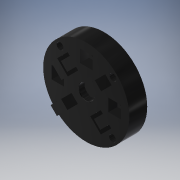
# Autodesk Inventor part: amt_socket
Saved by Autodesk Inventor 2019 (Build 230136000, 136)
## iProperties
Created: 2024-04-30
Part Number: amt_socket
Material: Acetalharz, Schwarz
Document SubType Name: Modeling
Designer: nic
Density: 1.425 g/cm^3
Appearance: Glatt - Schwarz
Author: nic
Autodesk Inventor part; units mm, degrees
ref_plane "YZ Plane" through (0, 0, 0) normal (1, 0, 0) x (0, 1, 0)
ref_plane "XZ Plane" through (0, 0, 0) normal (0, 1, 0) x (-1, 0, 0)
ref_plane "XY Plane" through (0, 0, 0) normal (0, 0, 1) x (1, 0, 0)
sketch "Skizze1" plane through (0, 0, 0) normal (0, 0, 1) x (1, 0, 0)
  circle A0 centre (0, 0) radius 14.5
  circle A1 centre (0, 0) radius 9.55 construction
  circle A2 centre (9.55, 0) radius 1.5
  circle A3 centre (-9.55, 0) radius 1.5
  circle A4 centre (0, 9.55) radius 1.5
  dimension "d0" = 29
  dimension "d1" = 19.1
  dimension "d2" = 3
  dimension "d3" = 3
  dimension "d4" = 3
  constraints: 5 centre point, 3 point on circle, 2 coincident
  measures "d0" diameter of A0
  measures "d1" diameter of A1
  measures "d2" diameter of A2
  measures "d3" diameter of A3
  measures "d4" diameter of A4
extrude "Extrusion1" add sketch "Skizze1" along normal blind 6
sketch "Skizze2" plane through (0, 0, 6) normal (0, 0, 1) x (1, 0, 0)
  circle A0 centre (0, 0) radius 5.6
  dimension "d7" = 11.2
  constraints: 1 centre point, 1 coincident
  measures "d7" diameter of A0
extrude "Extrusion2" cut sketch "Skizze2" against normal blind 5
sketch "Skizze3" plane through (0, 0, 1) normal (0, 0, 1) x (1, 0, 0)
  circle A0 centre (0, 0) radius 5.6 projected
  circle A1 centre (0, 0) radius 1.5
  dimension "d10" = 3
  constraints: 1 centre point, 1 coincident
  measures "d10" diameter of A1
extrude "Extrusion3" cut sketch "Skizze3" against normal through all contours A1
sketch "Skizze4" plane through (0, 0, 6) normal (0, 0, 1) x (1, 0, 0)
  circle A0 centre (0, 9.55) radius 1.5 construction
  circle A1 centre (9.55, 0) radius 1.5 construction
  circle A2 centre (-9.55, 0) radius 1.5 construction
  line L0 (-2.85, 12.4) -> (2.85, 12.4)
  line L1 (2.85, 12.4) -> (2.85, 6.7)
  line L2 (2.85, 6.7) -> (-2.85, 6.7)
  line L3 (-2.85, 6.7) -> (-2.85, 12.4)
  line L4 (-2.85, 12.4) -> (2.85, 6.7) construction
  line L5 (2.85, 12.4) -> (-2.85, 6.7) construction
  line L6 (-12.4, 2.85) -> (-6.7, 2.85)
  line L7 (-6.7, 2.85) -> (-6.7, -2.85)
  line L8 (-6.7, -2.85) -> (-12.4, -2.85)
  line L9 (-12.4, -2.85) -> (-12.4, 2.85)
  line L10 (-12.4, 2.85) -> (-6.7, -2.85) construction
  line L11 (-6.7, 2.85) -> (-12.4, -2.85) construction
  line L12 (6.7, 2.85) -> (12.4, 2.85)
  line L13 (12.4, 2.85) -> (12.4, -2.85)
  line L14 (12.4, -2.85) -> (6.7, -2.85)
  line L15 (6.7, -2.85) -> (6.7, 2.85)
  line L16 (6.7, 2.85) -> (12.4, -2.85) construction
  line L17 (12.4, 2.85) -> (6.7, -2.85) construction
  point P0 (0, 0)
  point P1 (9.55, 0)
  dimension "d13" = 5.7
  dimension "d14" = 5.7
  dimension "d15" = 5.7
  dimension "d16" = 5.7
  dimension "d17" = 5.7
  dimension "d18" = 5.7
  constraints: 36 end point, 6 midpoint, 6 parallel, 3 horizontal, 3 perpendicular
  measures "d13" distance of L1.end L2.end
  measures "d14" distance of L0.end L1.end
  measures "d15" distance of L7.end L8.end
  measures "d16" distance of L6.end L7.end
  measures "d17" distance of L13.end L14.end
  measures "d18" distance of L12.end L13.end
extrude "Extrusion4" cut sketch "Skizze4" against normal blind 3
sketch "Skizze5" plane through (0, 0, 6) normal (0, 0, 1) x (1, 0, 0)
  circle A0 centre (0, 0) radius 5.6 projected
  line L0 (0, -5.6) -> (0, -8.2) construction
  circle A1 centre (0, -8.2) radius 1.45
  dimension "d21" = 2.6
  dimension "d22" = 2.9
  constraints: 2 end point, 1 centre point, 1 coincident, 1 vertical, 1 vertical alignment, 1 other
  measures "d21" distance of L0.start L0.end
  measures "d22" diameter of A1
hole "Bohrung1" at (0, -8.2, 6) direction (0, 0, -1) diameter 2.9 end through all countersink diameter 6 countersink angle 90
sketch "Skizze6" plane through (0, 0, 6) normal (0, 0, 1) x (1, 0, 0)
  circle A0 centre (-8.8221, 9.0078) radius 2.6 construction
  circle A1 centre (-8.8221, 9.0078) radius 1.15
  circle A2 centre (-9.0078, -8.8221) radius 1.15
  circle A3 centre (8.8221, -9.0078) radius 1.15
  circle A4 centre (9.0078, 8.8221) radius 1.15
  point P0 (0, 0)
  dimension "d30" = 2.3
  dimension "d33" = 360
  constraints: 4 centre point, 1 coincident, 9 other
  measures "d30" diameter of A1
extrude "Extrusion5" cut sketch "Skizze6" against normal through all
sketch "Skizze7" plane through (0, 0, 6) normal (0, 0, 1) x (1, 0, 0)
  line L0 (-6.3847, -8.3956) -> (-2.8458, -4.8634)
  line L1 (-2.8458, -4.8634) -> (-4.9651, -2.7401)
  line L2 (-4.9651, -2.7401) -> (-8.504, -6.2723)
  line L3 (-8.504, -6.2723) -> (-6.3847, -8.3956)
  line L4 (-6.3847, -8.3956) -> (-4.9651, -2.7401) construction
  line L5 (-2.8458, -4.8634) -> (-8.504, -6.2723) construction
  line L6 (2.7401, -4.9651) -> (6.2723, -8.504)
  line L7 (6.2723, -8.504) -> (8.3956, -6.3847)
  line L8 (8.3956, -6.3847) -> (4.8634, -2.8458)
  line L9 (4.8634, -2.8458) -> (2.7401, -4.9651)
  line L10 (4.9651, 2.7401) -> (8.504, 6.2723)
  line L11 (8.504, 6.2723) -> (6.3847, 8.3956)
  line L12 (6.3847, 8.3956) -> (2.8458, 4.8634)
  line L13 (2.8458, 4.8634) -> (4.9651, 2.7401)
  line L14 (-2.7401, 4.9651) -> (-6.2723, 8.504)
  line L15 (-6.2723, 8.504) -> (-8.3956, 6.3847)
  line L16 (-8.3956, 6.3847) -> (-4.8634, 2.8458)
  line L17 (-4.8634, 2.8458) -> (-2.7401, 4.9651)
  point P0 (0, 0)
  point P1 (-5.6749, -5.5679)
  dimension "d37" = 5
  dimension "d38" = 3
  dimension "d41" = 360
  constraints: 36 end point, 2 midpoint, 2 parallel, 1 perpendicular, 33 other
  measures "d37" distance of L0.start L0.end
  measures "d38" distance of L1.end L0.end
extrude "Extrusion6" add sketch "Skizze7" along normal blind 3.5
sketch "Skizze8" plane through (-6.2723, 8.504, 9.5) normal (0.7077769, 0.706436, 0) x (0, 0, -1)
  line L0 (3.5, 0) -> (3.5, -5) projected
  line L1 (3.5, 0) -> (0, 0) projected
  line L2 (0, -5) -> (0, 0) projected
  line L3 (3.5, -5) -> (0, -5) projected
  line L4 (3.5, -4) -> (0.5, -4)
  line L5 (0.5, -4) -> (0.5, -1)
  line L6 (0.5, -1) -> (3.5, -1)
  line L7 (3.5, 4.0501) -> (3.5, -24.9499) projected
  line L8 (6.5, -4) -> (0.5, -1) construction
  line L9 (0.5, -4) -> (6.5, -1) construction
  line L10 (3.5, -3.6868) -> (3.5, -7.7212) projected
  line L11 (3.5, -4) -> (3.5, -1)
  line L12 (0.5, -4) -> (3.5, -4)
  line L13 (3.5, -4) -> (3.5, -1)
  line L14 (3.5, -1) -> (0.5, -1)
  line L15 (0.5, -1) -> (0.5, -4)
  point P0 (9.5, -10.4499)
  point P1 (3.5, -2.5)
  dimension "d46" = 3
  constraints: 20 end point, 3 parallel, 3 point on line, 2 horizontal, 2 midpoint, 2 perpendicular
  measures "d46" distance of L4.end L5.end
extrude "Extrusion7" cut sketch "Skizze8" against normal through all contours L0 L4 L5 L6
sketch "Skizze9" plane through (-8.504, -6.2723, 9.5) normal (-0.706436, 0.7077769, 0) x (0.7077769, 0.706436, 0)
  line L0 (0, 3.5) -> (5, 3.5) projected
  line L1 (0, 3.5) -> (0, 0) projected
  line L2 (5, 0) -> (0, 0) projected
  line L3 (5, 3.5) -> (5, 0) projected
  line L4 (-4.0501, 3.5) -> (24.9499, 3.5) projected
  line L5 (4.1701, 3.5) -> (1.1701, 3.5)
  line L6 (1.1701, 3.5) -> (1.1701, 0.5)
  line L7 (1.1701, 0.5) -> (4.1701, 0.5)
  line L8 (4.1701, 0.5) -> (4.1701, 3.5)
  point P0 (10.4499, 9.5)
  dimension "d49" = 3
  dimension "d50" = 3
  constraints: 8 end point, 2 parallel, 1 horizontal, 1 perpendicular, 1 point on line
  measures "d49" distance of L7.end L6.end
  measures "d50" distance of L6.end L5.end
extrude "Extrusion8" cut sketch "Skizze9" against normal through all contours L0 L8 L7 L6
sketch "Skizze10" plane through (6.2723, -8.504, 6) normal (-0.7077769, -0.706436, 0) x (0, 0, 1)
  line L0 (0, 0) -> (0, 5) projected
  line L1 (0, 0) -> (3.5, 0) projected
  line L2 (3.5, 5) -> (3.5, 0) projected
  line L3 (0, 5) -> (3.5, 5) projected
  line L4 (0, 0) -> (0, 5) projected
  line L5 (0, 4.0135) -> (3, 4.0135)
  line L6 (3, 4.0135) -> (3, 1.0135)
  line L7 (3, 1.0135) -> (0, 1.0135)
  line L8 (0, 1.0135) -> (0, 4.0135)
  point P0 (-6, 10.4499)
  dimension "d53" = 3
  dimension "d54" = 3
  constraints: 8 end point, 2 parallel, 1 horizontal, 1 perpendicular, 1 point on line
  measures "d53" distance of L6.end L7.end
  measures "d54" distance of L5.end L6.end
extrude "Extrusion9" cut sketch "Skizze10" against normal through all contours L0 L5 L6 L7
sketch "Skizze11" plane through (8.504, 6.2723, 6) normal (0.706436, -0.7077769, 0) x (0.7077769, 0.706436, 0)
  line L0 (-4.8499, 0) -> (-4.8499, -5) projected
  line L1 (0, 0) -> (-5, 0) projected
  line L2 (0, 0) -> (0, 3.5) projected
  line L3 (-5, 3.5) -> (0, 3.5) projected
  line L4 (-5, 0) -> (-5, 3.5) projected
  line L5 (-3.6996, 0) -> (-7.734, 0) projected
  line L6 (-3.942, 0) -> (-0.942, 0)
  line L7 (-0.942, 0) -> (-0.942, 3)
  line L8 (-0.942, 3) -> (-3.942, 3)
  line L9 (-3.942, 3) -> (-3.942, 0)
  point P0 (-10.4499, -6)
  dimension "d57" = 3
  dimension "d58" = 3
  constraints: 8 end point, 2 parallel, 1 horizontal, 1 perpendicular, 1 point on line
  measures "d57" distance of L8.end L7.end
  measures "d58" distance of L7.end L6.end
extrude "Extrusion10" cut sketch "Skizze11" against normal through all contours L1 L9 L8 L7
sketch "Skizze12" plane through (0, 0, 0) normal (0, 0, -1) x (-1, 0, 0)
  circle A0 centre (0, 0) radius 5.6 projected
  circle A1 centre (0, 0) radius 1.15
  dimension "d61" = 2.3
  constraints: 1 centre point, 1 coincident
  measures "d61" diameter of A1
extrude "Extrusion11" add sketch "Skizze12" against normal up to surface (6 mm away)
sketch "Skizze13" plane through (0, 0, 6) normal (0, 0, 1) x (1, 0, 0)
  circle A0 centre (0, 0) radius 1.15 projected
  circle A1 centre (0, 0) radius 2.6
  dimension "d64" = 5.2
  constraints: 1 centre point, 1 coincident
  measures "d64" diameter of A1
extrude "Extrusion12" cut sketch "Skizze13" against normal blind 2
sketch "Skizze14" plane through (0, 0, 0) normal (0, 0, -1) x (-1, 0, 0)
  circle A0 centre (0, 0) radius 2.6 projected
  circle A1 centre (0, 0) radius 1.15 projected
extrude "Extrusion13" cut sketch "Skizze14" against normal blind 2.5
sketch "Skizze15" plane through (0, 0, 6) normal (0, 0, 1) x (1, 0, 0)
  circle A0 centre (0, 0) radius 2.6 projected
  circle A1 centre (0, 0) radius 2.65
  dimension "d69" = 0.05
  constraints: 1 centre point
  measures "d69" radial gap between concentric circles of A0 A1
extrude "Extrusion14" cut sketch "Skizze15" against normal up to surface (2 mm away)
sketch "Skizze16" plane through (0, 0, 0) normal (0, 0, -1) x (-1, 0, 0)
  circle A0 centre (0, 0) radius 2.65 projected
extrude "Extrusion15" cut sketch "Skizze16" against normal up to surface (2.5 mm away)
sketch "Skizze17" plane through (0, 0, 6) normal (0, 0, 1) x (1, 0, 0)
  circle A0 centre (0, -8.2) radius 1.45 projected
  spline S0 degree 7 poles (1.2293, -5.4634) (1.147, -5.4819) (1.062, -5.4995) (0.9736, -5.5162) (0.8812, -5.5319) (0.7844, -5.5463) (0.6826, -5.5593) (0.5462, -5.5734) (0.5168, -5.5762) (0.4871, -5.5789) (0.4569, -5.5815) (0.4263, -5.5839) (0.3954, -5.5861) (0.3471, -5.5893) (0.3301, -5.5903) (0.3129, -5.5913) (0.2956, -5.5922) (0.2782, -5.5931) (0.2608, -5.594) (0.2093, -5.5962) (0.1751, -5.5974) (0.1406, -5.5984) (0.1059, -5.5992) (0.0711, -5.5997) (0.0362, -5.6) (-0.0517, -5.6) (-0.1047, -5.5994) (-0.1574, -5.5983) (-0.2096, -5.5966) (-0.2612, -5.5943) (-0.3119, -5.5915) (-0.3929, -5.5863) (-0.4239, -5.5841) (-0.4544, -5.5817) (-0.4846, -5.5792) (-0.5143, -5.5765) (-0.5437, -5.5736) (-0.6806, -5.5595) (-0.7828, -5.5466) (-0.88, -5.5321) (-0.9727, -5.5164) (-1.0614, -5.4997) (-1.1467, -5.482) (-1.2293, -5.4634) knots 0 0 0 0 0 0 0 0 0.294265 0.294265 0.294265 0.294265 0.294265 0.294265 0.373562 0.373562 0.373562 0.373562 0.373562 0.373562 0.416526 0.416526 0.416526 0.416526 0.416526 0.416526 0.499551 0.499551 0.499551 0.499551 0.499551 0.499551 0.625482 0.625482 0.625482 0.625482 0.625482 0.625482 0.70472 0.70472 0.70472 0.70472 0.70472 0.70472 1 1 1 1 1 1 1 1 projected
  arc A1 (-1.2293, -5.4634) -> (1.2293, -5.4634) centre (0, -8.2) ccw projected
  point P0 (0, 0)
  constraints: 1 horizontal alignment
extrude "Extrusion16" add sketch "Skizze17" against normal up to surface (6 mm away) contours A0 | A1 S0
sketch "Skizze18" plane through (0, 0, 6) normal (0, 0, 1) x (1, 0, 0)
  line L0 (-6.7, -2.85) -> (-12.4, -2.85) projected
  circle A0 centre (0, 0) radius 2.65 projected
  line L1 (4.9651, 2.7401) -> (2.8458, 4.8634) projected
  line L2 (2.8458, 4.8634) -> (3.5947, 5.6109) projected
  line L3 (5.714, 3.4875) -> (3.5947, 5.6109) projected
  line L4 (5.714, 3.4875) -> (4.9651, 2.7401) projected
  line L5 (2.7401, -4.9651) -> (4.8634, -2.8458) projected
  line L6 (4.8634, -2.8458) -> (5.5603, -3.5441) projected
  line L7 (3.437, -5.6634) -> (5.5603, -3.5441) projected
  line L8 (3.437, -5.6634) -> (2.7401, -4.9651) projected
  line L9 (-2.7401, 4.9651) -> (-4.8634, 2.8458) projected
  line L10 (-4.8634, 2.8458) -> (-5.5699, 3.5536) projected
  line L11 (-3.4465, 5.6729) -> (-5.5699, 3.5536) projected
  line L12 (-3.4465, 5.6729) -> (-2.7401, 4.9651) projected
  line L13 (-4.9651, -2.7401) -> (-2.8458, -4.8634) projected
  line L14 (-2.8458, -4.8634) -> (-3.4332, -5.4497) projected
  line L15 (-5.5525, -3.3264) -> (-3.4332, -5.4497) projected
  line L16 (-5.5525, -3.3264) -> (-4.9651, -2.7401) projected
  line L17 (7.8373, 5.6068) -> (5.718, 7.7302) projected
  line L18 (5.718, 7.7302) -> (6.3847, 8.3956) projected
  line L19 (6.3847, 8.3956) -> (8.504, 6.2723) projected
  line L20 (8.504, 6.2723) -> (7.8373, 5.6068) projected
  line L21 (2.85, 12.4) -> (2.85, 6.7) projected
  line L22 (2.85, 6.7) -> (-2.85, 6.7) projected
  line L23 (-2.85, 6.7) -> (-2.85, 12.4) projected
  line L24 (-2.85, 12.4) -> (2.85, 12.4) projected
  line L25 (-7.6759, -5.4457) -> (-5.5565, -7.569) projected
  line L26 (-5.5565, -7.569) -> (-6.3847, -8.3956) projected
  line L27 (-6.3847, -8.3956) -> (-8.504, -6.2723) projected
  line L28 (-8.504, -6.2723) -> (-7.6759, -5.4457) projected
  circle A1 centre (9.0078, 8.8221) radius 1.15 projected
  circle A2 centre (-9.0078, -8.8221) radius 1.15 projected
  circle A3 centre (-8.8221, 9.0078) radius 1.15 projected
  circle A4 centre (8.8221, -9.0078) radius 1.15 projected
  line L29 (-6.7, 2.85) -> (-6.7, -2.85) projected
  line L30 (-6.7, -2.85) -> (-12.4, -2.85) projected
  line L31 (-12.4, -2.85) -> (-12.4, 2.85) projected
  line L32 (-12.4, 2.85) -> (-6.7, 2.85) projected
  line L33 (-7.6892, 5.6769) -> (-8.3956, 6.3847) projected
  line L34 (-8.3956, 6.3847) -> (-6.2723, 8.504) projected
  line L35 (-6.2723, 8.504) -> (-5.5659, 7.7963) projected
  line L36 (-5.5659, 7.7963) -> (-7.6892, 5.6769) projected
  line L37 (12.4, -2.85) -> (6.7, -2.85) projected
  line L38 (6.7, -2.85) -> (6.7, 2.85) projected
  line L39 (6.7, 2.85) -> (12.4, 2.85) projected
  line L40 (12.4, 2.85) -> (12.4, -2.85) projected
  line L41 (5.5563, -7.7867) -> (7.6796, -5.6674) projected
  line L42 (7.6796, -5.6674) -> (8.3956, -6.3847) projected
  line L43 (8.3956, -6.3847) -> (6.2723, -8.504) projected
  line L44 (6.2723, -8.504) -> (5.5563, -7.7867) projected
  circle A5 centre (0, 0) radius 14.5 projected
  line L45 (-11.65, 2.1) -> (-11.65, -2.1)
  line L46 (-11.65, -2.1) -> (-7.45, -2.1)
  line L47 (-7.45, -2.1) -> (-7.45, 2.1)
  line L48 (-7.45, 2.1) -> (-11.65, 2.1)
  line L49 (2.1, 11.65) -> (2.1, 7.45)
  line L50 (2.1, 7.45) -> (-2.1, 7.45)
  line L51 (-2.1, 7.45) -> (-2.1, 11.65)
  line L52 (-2.1, 11.65) -> (2.1, 11.65)
  line L53 (7.45, 2.1) -> (7.45, -2.1)
  line L54 (7.45, -2.1) -> (11.65, -2.1)
  line L55 (11.65, -2.1) -> (11.65, 2.1)
  line L56 (11.65, 2.1) -> (7.45, 2.1)
  dimension "d76" = 0.75
  dimension "d77" = 0.75
  dimension "d78" = 0.75
  constraints: 24 end point, 9 other
  measures "d76" distance between parallel lines of L31 L45
  measures "d77" distance between parallel lines of L24 L52
  measures "d78" distance between parallel lines of L38 L53
extrude "Extrusion17" add sketch "Skizze18" against normal up to surface (3 mm away) contours L0 L31 L32 L29 | L21 L22 L23 L24 | L37 L38 L39 L40
sketch "Skizze19" plane through (0, 0, 4) normal (0, 0, 1) x (1, 0, 0)
  circle A0 centre (0, 0) radius 1.15 projected
  circle A1 centre (0, 0) radius 1.45
  dimension "d81" = 0.3
  constraints: 1 centre point
  measures "d81" radial gap between concentric circles of A0 A1
extrude "Extrusion18" cut sketch "Skizze19" against normal through all
sketch "Skizze20" plane through (0, 0, 6) normal (0, 0, 1) x (1, 0, 0)
  circle A0 centre (0, 0) radius 2.65 projected
  circle A1 centre (0, 0) radius 2.575
  dimension "d90" = 0.075
  constraints: 1 centre point
  measures "d90" radial gap between concentric circles of A0 A1
extrude "Extrusion19" add sketch "Skizze20" against normal up to surface (6 mm away)
chamfer "Fase3" distance 0.1 angle 45 2 edges at (-2.575, 0, 0) (-2.575, 0, 6)
